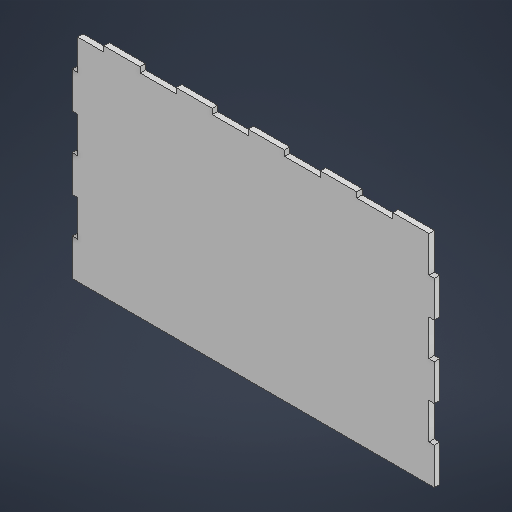
# Autodesk Inventor part: Part2
Saved by Autodesk Inventor 2027.1 (Build 311270010, 270A)
## iProperties
Created: 2026-10-07
Part Number: Part2
Material: Generic
Document SubType Name: Modeling
Designer: daniel
Density: 1 g/cm^3
Appearance: Default
Mass: 70.0785 g
Surface Area: 487.83 cm^2
Volume: 70.0785 cm^3
Author: daniel
Autodesk Inventor part; units mm, degrees
ref_plane "YZ Plane" through (0, 0, 0) normal (1, 0, 0) x (0, 1, 0)
ref_plane "XZ Plane" through (0, 0, 0) normal (0, 1, 0) x (-1, 0, 0)
ref_plane "XY Plane" through (0, 0, 0) normal (0, 0, 1) x (1, 0, 0)
sketch "Sketch1" plane through (0, 0, 0) normal (0, 0, 1) x (1, 0, 0)
  line L0 (26.7826, 135.7478) -> (226.7826, 135.7478)
  line L1 (226.7826, 135.7478) -> (226.7826, 15.7478)
  line L2 (226.7826, 15.7478) -> (26.7826, 15.7478)
  line L3 (26.7826, 15.7478) -> (26.7826, 135.7478)
  line L4 (26.7826, 135.7478) -> (29.7826, 135.7478)
  line L5 (29.7826, 135.7478) -> (29.7826, 115.8478)
  line L6 (29.7826, 115.8478) -> (26.7826, 115.8478)
  line L7 (26.7826, 115.8478) -> (26.7826, 135.7478)
  line L8 (29.7826, 115.8478) -> (26.7826, 115.8478)
  line L9 (26.7826, 115.8478) -> (26.7826, 95.8478)
  line L10 (26.7826, 95.8478) -> (29.7826, 95.8478)
  line L11 (29.7826, 95.8478) -> (29.7826, 115.8478)
  line L12 (26.7826, 95.8478) -> (29.7826, 95.8478)
  line L13 (29.7826, 95.8478) -> (29.7826, 75.9478)
  line L14 (29.7826, 75.9478) -> (26.7826, 75.9478)
  line L15 (26.7826, 75.9478) -> (26.7826, 95.8478)
  line L16 (29.7826, 75.9478) -> (26.7826, 75.9478)
  line L17 (26.7826, 75.9478) -> (26.7826, 55.9478)
  line L18 (26.7826, 55.9478) -> (29.7826, 55.9478)
  line L19 (29.7826, 55.9478) -> (29.7826, 75.9478)
  line L20 (29.7826, 55.9478) -> (26.7826, 55.9478)
  line L21 (26.7826, 55.9478) -> (26.7826, 36.0478)
  line L22 (26.7826, 36.0478) -> (29.7826, 36.0478)
  line L23 (29.7826, 36.0478) -> (29.7826, 55.9478)
  line L24 (26.7826, 36.0478) -> (29.7826, 36.0478)
  line L25 (29.7826, 36.0478) -> (29.7826, 15.7478)
  line L26 (29.7826, 15.7478) -> (26.7826, 15.7478)
  line L27 (26.7826, 15.7478) -> (26.7826, 36.0478)
  line L28 (126.7826, 150.5528) -> (126.7826, -31.6323)
  line L29 (226.7826, 15.7478) -> (226.7826, 135.7478)
  line L30 (226.7826, 135.7478) -> (223.7826, 135.7478)
  line L31 (223.7826, 135.7478) -> (223.7826, 115.8478)
  line L32 (223.7826, 115.8478) -> (226.7826, 115.8478)
  line L33 (226.7826, 115.8478) -> (226.7826, 135.7478)
  line L34 (223.7826, 115.8478) -> (226.7826, 115.8478)
  line L35 (226.7826, 115.8478) -> (226.7826, 95.8478)
  line L36 (226.7826, 95.8478) -> (223.7826, 95.8478)
  line L37 (223.7826, 95.8478) -> (223.7826, 115.8478)
  line L38 (226.7826, 95.8478) -> (223.7826, 95.8478)
  line L39 (223.7826, 95.8478) -> (223.7826, 75.9478)
  line L40 (223.7826, 75.9478) -> (226.7826, 75.9478)
  line L41 (226.7826, 75.9478) -> (226.7826, 95.8478)
  line L42 (223.7826, 75.9478) -> (226.7826, 75.9478)
  line L43 (226.7826, 75.9478) -> (226.7826, 55.9478)
  line L44 (226.7826, 55.9478) -> (223.7826, 55.9478)
  line L45 (223.7826, 55.9478) -> (223.7826, 75.9478)
  line L46 (223.7826, 55.9478) -> (226.7826, 55.9478)
  line L47 (226.7826, 55.9478) -> (226.7826, 36.0478)
  line L48 (226.7826, 36.0478) -> (223.7826, 36.0478)
  line L49 (223.7826, 36.0478) -> (223.7826, 55.9478)
  line L50 (226.7826, 36.0478) -> (223.7826, 36.0478)
  line L51 (223.7826, 36.0478) -> (223.7826, 15.7478)
  line L52 (223.7826, 15.7478) -> (226.7826, 15.7478)
  line L53 (226.7826, 15.7478) -> (226.7826, 36.0478)
  line L54 (223.7826, 135.7478) -> (203.7826, 135.7478)
  line L55 (203.7826, 135.7478) -> (203.7826, 132.7478)
  line L56 (203.7826, 132.7478) -> (223.7826, 132.7478)
  line L57 (223.7826, 132.7478) -> (223.7826, 135.7478)
  line L58 (203.7826, 132.7478) -> (183.8826, 132.7478)
  line L59 (183.8826, 132.7478) -> (183.8826, 135.7478)
  line L60 (183.8826, 135.7478) -> (203.7826, 135.7478)
  line L61 (203.7826, 135.7478) -> (203.7826, 132.7478)
  line L62 (183.8826, 132.7478) -> (163.8826, 132.7478)
  line L63 (163.8826, 132.7478) -> (163.8826, 135.7478)
  line L64 (163.8826, 135.7478) -> (183.8826, 135.7478)
  line L65 (183.8826, 135.7478) -> (183.8826, 132.7478)
  line L66 (163.8826, 132.7478) -> (143.9826, 132.7478)
  line L67 (143.9826, 132.7478) -> (143.9826, 135.7478)
  line L68 (143.9826, 135.7478) -> (163.8826, 135.7478)
  line L69 (163.8826, 135.7478) -> (163.8826, 132.7478)
  line L70 (143.9826, 132.7478) -> (123.9826, 132.7478)
  line L71 (123.9826, 132.7478) -> (123.9826, 135.7478)
  line L72 (123.9826, 135.7478) -> (143.9826, 135.7478)
  line L73 (143.9826, 135.7478) -> (143.9826, 132.7478)
  line L74 (123.9826, 132.7478) -> (104.0826, 132.7478)
  line L75 (104.0826, 132.7478) -> (104.0826, 135.7478)
  line L76 (104.0826, 135.7478) -> (123.9826, 135.7478)
  line L77 (123.9826, 135.7478) -> (123.9826, 132.7478)
  line L78 (104.0826, 132.7478) -> (29.7826, 132.7478)
  line L79 (29.7826, 132.7478) -> (29.7826, 135.7478)
  line L80 (29.7826, 135.7478) -> (104.0826, 135.7478)
  line L81 (104.0826, 135.7478) -> (104.0826, 132.7478)
  line L82 (104.1826, 135.7478) -> (104.1826, 132.7478)
  line L83 (104.1826, 132.7478) -> (84.1826, 132.7478)
  line L84 (84.1826, 132.7478) -> (84.1826, 135.7478)
  line L85 (84.1826, 135.7478) -> (104.1826, 135.7478)
  line L86 (104.1826, 135.7478) -> (104.1826, 132.7478)
  line L87 (84.1826, 132.7478) -> (64.2826, 132.7478)
  line L88 (64.2826, 132.7478) -> (64.2826, 135.7478)
  line L89 (64.2826, 135.7478) -> (84.1826, 135.7478)
  line L90 (84.1826, 135.7478) -> (84.1826, 132.7478)
  line L91 (64.2826, 132.7478) -> (44.2826, 132.7478)
  line L92 (44.2826, 132.7478) -> (44.2826, 135.7478)
  line L93 (44.2826, 135.7478) -> (64.2826, 135.7478)
  line L94 (64.2826, 135.7478) -> (64.2826, 132.7478)
  line L95 (44.2826, 135.7478) -> (44.2826, 132.7478)
  point P0 (0, 0)
  point P1 (29.7826, 95.8478)
  point P2 (26.7826, 75.9478)
  point P3 (226.7826, 36.0478)
  point P4 (226.7826, 55.9478)
  point P5 (226.7826, 75.9478)
  point P6 (223.7826, 95.8478)
  point P7 (226.7826, 95.8478)
  point P8 (226.7826, 115.8478)
  point P9 (223.7826, 135.7478)
  point P10 (26.7826, 115.8478)
  point P11 (26.7826, 95.8478)
  point P12 (203.7826, 135.7478)
  point P13 (225.2826, 135.7478)
  point P14 (225.2826, 115.8478)
  point P15 (225.2826, 115.8478)
  point P16 (225.2826, 95.8478)
  point P17 (27.0826, 150.5528)
  dimension "d0" = 200
  dimension "d1" = 120
  dimension "d2" = 3
  dimension "d3" = 19.9
  dimension "d4" = 20
  dimension "d5" = 3
  dimension "d6" = 19.9
  dimension "d7" = 20
  dimension "d8" = 19.9
  dimension "d11" = 20
  dimension "d12" = 3
  dimension "d13" = 19.9
  dimension "d14" = 20
  dimension "d15" = 19.9
  dimension "d16" = 20
  dimension "d17" = 19.9
  dimension "d18" = 19.9
  dimension "d19" = 20
  dimension "d20" = 3
  dimension "d21" = 20
  dimension "d22" = 19.9
  dimension "d23" = 20
  constraints: 192 end point, 34 parallel, 19 symmetric about line, 17 horizontal, 17 perpendicular, 12 point on line, 4 midpoint, 1 vertical
  measures "d0" distance of L1.end L2.end
  measures "d1" distance of L0.end L1.end
  measures "d2" distance of L5.end L6.end
  measures "d3" distance of L4.end L5.end
  measures "d4" distance of L9.end L8.end
  measures "d5" distance between parallel lines of L11 L9
  measures "d6" distance of L12.end L13.end
  measures "d7" distance of L17.end L16.end
  measures "d8" distance of L21.end L20.end
  measures "d11" distance of L56.end L55.end
  measures "d12" distance of L55.end L54.end
  measures "d13" distance of L59.end L60.end
  measures "d14" distance of L63.end L64.end
  measures "d15" distance of L67.end L68.end
  measures "d16" distance of L71.end L72.end
  measures "d17" distance of L75.end L76.end
  measures "d18" distance of point (225.283, 135.748) point (225.283, 115.848)
  measures "d19" distance of point (225.283, 115.848) point (225.283, 95.848)
  measures "d20" distance of L83.start L82.start
  measures "d21" distance of L85.start L86.start
  measures "d22" distance of L88.end L89.end
  measures "d23" distance of L93.start L93.end
extrude "Extrusion1" add sketch "Sketch1" along normal blind 3 contours L6 L11 L10 L3 | L0 L88 L78 L92 | L78 L74 L70 L28 L2 L25 L23 L19 L13 L11 L5 | L14 L19 L18 L3 | L0 L75 L78 L84 | L22 L25 L2 L3 | L0 L28 L70 L71 | L0 L67 L70 L28 | L28 L70 L66 L62 L58 L56 L31 L37 L39 L45 L49 L51 L2 | L51 L48 L1 L2 | L0 L59 L62 L63 | L45 L40 L1 L44 | L0 L31 L56 L55 | L37 L32 L1 L36
equation "\"d3\" = d6"
equation "\"d8\" = d6"
equation "\"d13\" = d6"
equation "\"d15\" = d3"
equation "\"d17\" = d3"
equation "\"d27\" = d26"
equation "\"d26\" = 19.9"
body "Solid1"
